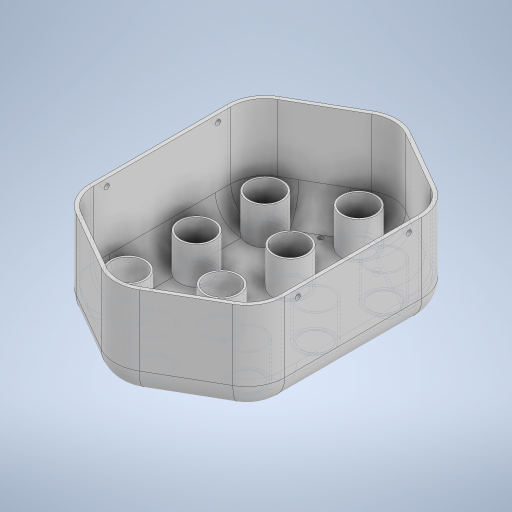
# Autodesk Inventor part: Caixa_10_amostras_v2
Saved by Autodesk Inventor 2024 (Build 280153000, 153)
## iProperties
Created: 2025-07-22
Part Number: Caixa_10_amostras_v2
Material: Generic
Document SubType Name: Modeling
Designer: Bruno
Density: 1 g/cm^3
Appearance: Default
Author: Bruno
Autodesk Inventor part; units mm, degrees
ref_plane "YZ Plane" through (0, 0, 0) normal (1, 0, 0) x (0, 1, 0)
ref_plane "XZ Plane" through (0, 0, 0) normal (0, 1, 0) x (-1, 0, 0)
ref_plane "XY Plane" through (0, 0, 0) normal (0, 0, 1) x (1, 0, 0)
sketch "Sketch1" plane through (0, 0, 0) normal (0, 1, 0) x (-1, 0, 0)
  line L0 (100, -100) -> (-100, -100)
  line L1 (-100, -100) -> (-100, 100)
  line L2 (-100, 100) -> (100, 100)
  line L3 (100, 100) -> (100, -100)
  line L4 (100, -100) -> (-100, 100)
  point P0 (0, 0)
  point P1 (0, 0)
  dimension "d0" = 200
  dimension "d1" = 200
  constraints: 10 end point, 2 parallel, 1 coincident, 1 horizontal, 1 midpoint, 1 perpendicular
  measures "d0" distance of L0.end L1.end
  measures "d1" distance of L0.start L0.end
extrude "Extrusion1" add sketch "Sketch1" along normal blind 2
sketch "Sketch2" plane through (0, 2, 0) normal (0, 1, 0) x (1, 0, 0)
  line L0 (100, 100) -> (-100, 100)
  line L1 (0, 100) -> (0, -100)
  line L2 (-100, -100) -> (100, -100)
  line L3 (100, -100) -> (100, 100)
  line L4 (100, 0) -> (-100, 0)
  line L5 (-100, 100) -> (-100, -100)
  circle A0 centre (0, -55.5) radius 18.5
  circle A1 centre (0, -55.5) radius 8.5
  circle A2 centre (0, -55.5) radius 17.5
  circle A3 centre (0, -55.5) radius 7.5
  circle A4 centre (0, -18.5) radius 7.5
  circle A5 centre (0, -18.5) radius 8.5
  circle A6 centre (0, -18.5) radius 17.5
  circle A7 centre (0, -18.5) radius 18.5
  circle A8 centre (0, 18.5) radius 7.5
  circle A9 centre (0, 18.5) radius 8.5
  circle A10 centre (0, 18.5) radius 17.5
  circle A11 centre (0, 18.5) radius 18.5
  circle A12 centre (0, 55.5) radius 7.5
  circle A13 centre (0, 55.5) radius 8.5
  circle A14 centre (0, 55.5) radius 17.5
  circle A15 centre (0, 55.5) radius 18.5
  circle A16 centre (-32.04294, -37) radius 7.5
  circle A17 centre (-32.04294, -37) radius 8.5
  circle A18 centre (-32.04294, -37) radius 17.5
  circle A19 centre (-32.04294, -37) radius 18.5
  circle A20 centre (-32.04294, 0) radius 7.5
  circle A21 centre (-32.04294, 0) radius 8.5
  circle A22 centre (-32.04294, 0) radius 17.5
  circle A23 centre (-32.04294, 0) radius 18.5
  circle A24 centre (-32.04294, 37) radius 7.5
  circle A25 centre (-32.04294, 37) radius 8.5
  circle A26 centre (-32.04294, 37) radius 17.5
  circle A27 centre (-32.04294, 37) radius 18.5
  circle A28 centre (32.05706, -37) radius 7.5
  circle A29 centre (32.05706, -37) radius 8.5
  circle A30 centre (32.05706, -37) radius 17.5
  circle A31 centre (32.05706, -37) radius 18.5
  circle A32 centre (32.05706, 0) radius 7.5
  circle A33 centre (32.05706, 0) radius 8.5
  circle A34 centre (32.05706, 0) radius 17.5
  circle A35 centre (32.05706, 0) radius 18.5
  circle A36 centre (32.05706, 37) radius 7.5
  circle A37 centre (32.05706, 37) radius 8.5
  circle A38 centre (32.05706, 37) radius 17.5
  circle A39 centre (32.05706, 37) radius 18.5
  point P0 (0, 0)
  point P1 (-32.04294, 18.5)
  point P2 (-16.02147, 27.75)
  point P3 (-16.02147, 46.25)
  point P4 (-16.02147, 9.25)
  point P5 (-32.04294, -18.5)
  point P6 (-16.02147, -9.25)
  point P7 (0, 37)
  point P8 (0, 0)
  point P9 (-16.02147, -27.75)
  point P10 (32.05706, 18.5)
  point P11 (32.05706, -18.5)
  dimension "d4" = 37
  dimension "d5" = 17
  dimension "d18" = 35
  dimension "d19" = 15
  dimension "d42" = 37
  dimension "d47" = 111
  dimension "d48" = 35
  dimension "d49" = 37
  dimension "d50" = 15
  dimension "d51" = 17
  dimension "d55" = 37
  dimension "d58" = 64.1
  constraints: 40 centre point, 30 coincident, 4 end point, 4 midpoint, 2 equal radius, 2 vertical, 1 horizontal, 1 point on line, 64 other
  measures "d4" diameter of A0
  measures "d5" diameter of A1
  measures "d18" diameter of A2
  measures "d19" diameter of A3
  measures "d42" distance of A3.centre A4.centre
  measures "d47" diameter of A0.centre L4
  measures "d48" diameter of A18
  measures "d49" diameter of A19
  measures "d50" diameter of A16
  measures "d51" diameter of A17
  measures "d55" distance of A16.centre A20.centre
  measures "d58" distance of A16.centre A28.centre
extrude "Extrusion2" cut sketch "Sketch2" against normal blind 0.1 contours A39 | A31 | A15 L1 A14 | L1 A14 A15 | A35 L4 A34 | L4 A34 A35 | A27 | A23 L4 A22 | L4 A22 A23 | A13 L1 A12 | L1 A12 A13 | A11 L1 A10 | L1 A10 A11 | A0 L1 A2 | L1 A2 A0 | A33 L4 A32 | L4 A32 A33 | A19 | A7 L1 A6 | L1 A6 A7 | A21 L4 A20 | L4 A20 A21 | A9 L1 A8 | L1 A8 A9 | A1 L1 A3 | L1 A3 A1 | A5 L1 A4 | L1 A4 A5 | A17 | A25 | A29 | A37
sketch "Sketch4" plane through (0, 2, 0) normal (0, 1, 0) x (1, 0, 0)
  arc A0 (-16.02147, 46.25) -> (-32.04294, 18.5) centre (-32.04294, 37) ccw
  line L0 (-41.29294, 53.02147) -> (-9.25, 71.52147)
  arc A1 (0, 37) -> (-16.02147, 46.25) centre (0, 55.5) ccw
  line L1 (9.246944, 71.523234) -> (41.304004, 53.023234)
  circle A2 centre (32.05706, 37) radius 18.5
  line L2 (50.55706, 37) -> (50.55706, -37)
  circle A3 centre (32.05706, -37) radius 18.5
  line L3 (41.304004, -53.023234) -> (9.246944, -71.523234)
  arc A4 (-16.02147, -46.25) -> (0, -37) centre (0, -55.5) ccw
  line L4 (-9.25, -71.52147) -> (-41.29294, -53.02147)
  line L5 (-50.54294, 37) -> (-50.54294, -37)
  arc A5 (-32.04294, -18.5) -> (-16.02147, -46.25) centre (-32.04294, -37) ccw
  line L6 (-100, 100) -> (-100, -100)
  line L7 (100, 100) -> (-100, 100)
  line L8 (100, -100) -> (100, 100)
  line L9 (-100, -100) -> (100, -100)
  point P0 (0, 0)
  point P1 (32.05706, 18.5)
  point P2 (32.05706, -18.5)
  constraints: 12 end point, 12 point on circle, 12 tangent
extrude "Extrusion4" cut sketch "Sketch4" against normal through all
sketch "Sketch6" plane through (0, 0, 0) normal (0, -1, 0) x (1, 0, 0)
  arc A0 (50.55706, 37) -> (41.304004, 53.023234) centre (32.05706, 37) ccw
  line L0 (41.304004, 53.023234) -> (9.246944, 71.523234)
  arc A1 (9.246944, 71.523234) -> (-9.25, 71.52147) centre (0, 55.5) ccw
  line L1 (-9.25, 71.52147) -> (-41.29294, 53.02147)
  arc A2 (-41.29294, 53.02147) -> (-50.54294, 37) centre (-32.04294, 37) ccw
  line L2 (-50.54294, 37) -> (-50.54294, -37)
  arc A3 (-50.54294, -37) -> (-41.29294, -53.02147) centre (-32.04294, -37) ccw
  line L3 (-41.29294, -53.02147) -> (-9.25, -71.52147)
  arc A4 (-9.25, -71.52147) -> (9.246944, -71.523234) centre (0, -55.5) ccw
  line L4 (9.246944, -71.523234) -> (41.304004, -53.023234)
  arc A5 (41.304004, -53.023234) -> (50.55706, -37) centre (32.05706, -37) ccw
  line L5 (50.55706, -37) -> (50.55706, 37)
  line L6 (10.246613, 73.255476) -> (42.303673, 54.755476)
  arc A6 (52.55706, 37) -> (42.303673, 54.755476) centre (32.05706, 37) ccw
  line L7 (52.55706, 37) -> (52.55706, -37)
  arc A7 (42.303673, -54.755476) -> (52.55706, -37) centre (32.05706, -37) ccw
  line L8 (42.303673, -54.755476) -> (10.246613, -73.255476)
  arc A8 (-10.25, -73.253521) -> (10.246613, -73.255476) centre (0, -55.5) ccw
  line L9 (-10.25, -73.253521) -> (-42.29294, -54.753521)
  arc A9 (-52.54294, -37) -> (-42.29294, -54.753521) centre (-32.04294, -37) ccw
  line L10 (-52.54294, -37) -> (-52.54294, 37)
  arc A10 (-42.29294, 54.753521) -> (-52.54294, 37) centre (-32.04294, 37) ccw
  line L11 (-42.29294, 54.753521) -> (-10.25, 73.253521)
  arc A11 (10.246613, 73.255476) -> (-10.25, 73.253521) centre (0, 55.5) ccw
  point P0 (0, 0)
  dimension "d65" = 2
  constraints: 12 end point, 12 point on circle, 6 centre point, 11 other
  measures "d65" distance between parallel lines of L6 L0
extrude "Extrusion6" add sketch "Sketch6" against normal blind 52
sketch "Sketch7" plane through (0, 1.9, 0) normal (0, 1, 0) x (1, 0, 0)
  arc A0 (-16.02147, -46.25) -> (-16.02147, -27.75) centre (-32.04294, -37) ccw
  arc A1 (-16.02147, -27.75) -> (-32.04294, -18.5) centre (-32.04294, -37) ccw
  arc A2 (-32.04294, -18.5) -> (-16.02147, -46.25) centre (-32.04294, -37) ccw
  circle A3 centre (-32.04294, -37) radius 17.5
  arc A4 (-16.02147, -9.25) -> (-16.02147, 9.25) centre (-32.04294, 0) ccw
  arc A5 (-16.02147, 9.25) -> (-32.04294, 18.5) centre (-32.04294, 0) ccw
  arc A6 (-32.04294, 18.5) -> (-32.04294, -18.5) centre (-32.04294, 0) ccw
  arc A7 (-32.04294, -18.5) -> (-16.02147, -9.25) centre (-32.04294, 0) ccw
  circle A8 centre (-32.04294, 0) radius 17.5
  arc A9 (-16.02147, 27.75) -> (-16.02147, 46.25) centre (-32.04294, 37) ccw
  arc A10 (-16.02147, 46.25) -> (-32.04294, 18.5) centre (-32.04294, 37) ccw
  arc A11 (-32.04294, 18.5) -> (-16.02147, 27.75) centre (-32.04294, 37) ccw
  circle A12 centre (-32.04294, 37) radius 17.5
  arc A13 (-16.02147, 46.25) -> (0, 37) centre (0, 55.5) ccw
  arc A14 (0, 37) -> (-16.02147, 46.25) centre (0, 55.5) ccw
  circle A15 centre (0, 55.5) radius 17.5
  arc A16 (-16.02147, 9.25) -> (0, 0) centre (0, 18.5) ccw
  arc A17 (0, 0) -> (0, 37) centre (0, 18.5) ccw
  arc A18 (0, 37) -> (-16.02147, 27.75) centre (0, 18.5) ccw
  arc A19 (-16.02147, 27.75) -> (-16.02147, 9.25) centre (0, 18.5) ccw
  circle A20 centre (0, 18.5) radius 17.5
  arc A21 (-16.02147, -9.25) -> (-16.02147, -27.75) centre (0, -18.5) ccw
  arc A22 (-16.02147, -27.75) -> (0, -37) centre (0, -18.5) ccw
  arc A23 (0, -37) -> (0, 0) centre (0, -18.5) ccw
  arc A24 (0, 0) -> (-16.02147, -9.25) centre (0, -18.5) ccw
  circle A25 centre (0, -18.5) radius 17.5
  arc A26 (-16.02147, -46.25) -> (0, -37) centre (0, -55.5) ccw
  arc A27 (0, -37) -> (-16.02147, -46.25) centre (0, -55.5) ccw
  circle A28 centre (0, -55.5) radius 17.5
  circle A29 centre (32.05706, -37) radius 18.5
  circle A30 centre (32.05706, -37) radius 17.5
  arc A31 (32.05706, -18.5) -> (32.05706, 18.5) centre (32.05706, 0) ccw
  arc A32 (32.05706, 18.5) -> (32.05706, -18.5) centre (32.05706, 0) ccw
  circle A33 centre (32.05706, 0) radius 17.5
  circle A34 centre (32.05706, 37) radius 18.5
  circle A35 centre (32.05706, 37) radius 17.5
  point P0 (0, 0)
  point P1 (32.05706, 18.5)
  point P2 (32.05706, 18.5)
  point P3 (32.05706, -18.5)
  point P4 (32.05706, -18.5)
  point P5 (0, 37)
  point P6 (0, 37)
  point P7 (0, 37)
  point P8 (0, 37)
  point P9 (-16.02147, 46.25)
  point P10 (-16.02147, 46.25)
  point P11 (-16.02147, 46.25)
  point P12 (-16.02147, 46.25)
  point P13 (-16.02147, 27.75)
  point P14 (-16.02147, 27.75)
  point P15 (-16.02147, 27.75)
  point P16 (-16.02147, 27.75)
  point P17 (0, -37)
  point P18 (0, -37)
  point P19 (0, -37)
  point P20 (0, -37)
  point P21 (-16.02147, -46.25)
  point P22 (-16.02147, -46.25)
  point P23 (-16.02147, -46.25)
  point P24 (-16.02147, -46.25)
  point P25 (-16.02147, -27.75)
  point P26 (-16.02147, -27.75)
  point P27 (-16.02147, -27.75)
  point P28 (-16.02147, -27.75)
  point P29 (-32.04294, -18.5)
  point P30 (-32.04294, -18.5)
  point P31 (-32.04294, -18.5)
  point P32 (-32.04294, -18.5)
  point P33 (0, 0)
  point P34 (0, 0)
  point P35 (0, 0)
  point P36 (0, 0)
  point P37 (-16.02147, -9.25)
  point P38 (-16.02147, -9.25)
  point P39 (-16.02147, -9.25)
  point P40 (-16.02147, -9.25)
  point P41 (-16.02147, 9.25)
  point P42 (-16.02147, 9.25)
  point P43 (-16.02147, 9.25)
  point P44 (-16.02147, 9.25)
  constraints: 2 other
extrude "Extrusion7" add sketch "Sketch7" along normal up to surface (0.1 mm away) contours A2 A1 A0 | A27 A26 | A21 A24 A23 A22 | A6 A5 A4 A7 | A10 A9 A11 | A16 A19 A18 A17 | A14 A13 | A29 | A34 | A32 A31
sketch "Sketch5" plane through (0, 2, -18.5) normal (0, 1, 0) x (1, 0, 0)
  circle A0 centre (-32.04294, 18.5) radius 8.5
  circle A1 centre (0, 37) radius 8.5
  circle A2 centre (32.05706, 18.5) radius 8.5
  circle A3 centre (0, 0) radius 8.5
  circle A4 centre (32.05706, -18.5) radius 8.5
  circle A5 centre (32.05706, -55.5) radius 8.5
  circle A6 centre (0, -37) radius 8.5
  circle A7 centre (0, -74) radius 8.5
  circle A8 centre (-32.04294, -55.5) radius 8.5
  circle A9 centre (-32.04294, -18.5) radius 8.5
  circle A10 centre (-32.04294, -55.5) radius 7.5
  circle A11 centre (-32.04294, -55.5) radius 9.5
  circle A12 centre (-32.04294, -18.5) radius 9.5
  circle A13 centre (-32.04294, 18.5) radius 9.5
  circle A14 centre (0, 0) radius 9.5
  circle A15 centre (0, 37) radius 9.5
  circle A16 centre (0, -37) radius 9.5
  circle A17 centre (0, -74) radius 9.5
  circle A18 centre (32.05706, -55.5) radius 9.5
  circle A19 centre (32.05706, -18.5) radius 9.5
  circle A20 centre (32.05706, 18.5) radius 7.5
  circle A21 centre (32.05706, 18.5) radius 9.5
  point P0 (0, -18.5)
  dimension "d68" = 1
  dimension "d69" = 1
  dimension "d70" = 1
  dimension "d71" = 1
  dimension "d72" = 1
  dimension "d73" = 1
  dimension "d74" = 1
  dimension "d75" = 1
  dimension "d76" = 1
  dimension "d77" = 1
  constraints: 10 centre point, 10 coincident
  measures "d68" radial gap between concentric circles of A11 A8
  measures "d69" radial gap between concentric circles of A12 A9
  measures "d70" radial gap between concentric circles of A13 A0
  measures "d71" radial gap between concentric circles of A16 A6
  measures "d72" radial gap between concentric circles of A14 A3
  measures "d73" radial gap between concentric circles of A15 A1
  measures "d74" radial gap between concentric circles of A17 A7
  measures "d75" radial gap between concentric circles of A18 A5
  measures "d76" radial gap between concentric circles of A19 A4
  measures "d77" radial gap between concentric circles of A21 A2
extrude "Extrusion5" add sketch "Sketch5" along normal blind 20 contours A11 | A12 | A13 | A14 | A15 | A16 | A17 | A18 | A19 | A21
fillet "Fillet2" radius 14 24 edges at (-48.0644, 2, 46.25) (-25.2715, 2, 62.2715) (-0.0018, 2, 74) (25.2755, 2, 62.2732) (48.0776, 2, 46.2515) (50.5571, 2, 0) (48.0776, 2, -46.2515) (25.2755, 2, -62.2732) (-0.0018, 2, -74) (-25.2715, 2, -62.2715) (-48.0644, 2, -46.25) (-50.5429, 2, 0) (49.8096, 0, 47.2517) (26.2751, 0, 64.0055) (-0.002, 0, 76) (-26.2715, 0, 64.0035) (-49.7965, 0, 47.25) (-52.5429, 0, 0) (-49.7965, 0, -47.25) (-26.2715, 0, -64.0035) (-0.002, 0, -76) (26.2751, 0, -64.0055) (49.8096, 0, -47.2517) (52.5571, 0, 0)
sketch "Sketch8" plane through (52.55706, 52, 37) normal (1, 0, 0) x (0, 0, -1)
  line L0 (37, 17.918603) -> (37, -112.555853)
  circle A0 centre (7, -3.9) radius 1.35
  line L1 (0, 0) -> (74, 0)
  circle A1 centre (67, -3.9) radius 1.35
  point P0 (37, -52)
  dimension "d81" = 2.7
  dimension "d82" = 60
  dimension "d83" = 3.9
  constraints: 2 centre point, 2 end point, 1 point on line, 1 symmetric about line, 1 vertical, 1 other
  measures "d81" diameter of A0
  measures "d82" diameter of A0.centre L0
  measures "d83" distance from line of L1 A0.centre
extrude "Extrusion8" cut sketch "Sketch8" against normal through all
sketch "Sketch9" plane through (0, 0, 0) normal (0, -1, 0) x (1, 0, 0)
  line L0 (-59.157848, 0) -> (59.157848, 0)
  line L1 (0, 117.504066) -> (0, -117.504066)
  circle A0 centre (-15, 50) radius 1.35
  circle A1 centre (15, 50) radius 1.35
  circle A2 centre (-15, -50) radius 1.35
  circle A3 centre (15, -50) radius 1.35
  point P0 (0, 0)
  point P1 (0, 0)
  dimension "d86" = 2.7
  dimension "d87" = 100
  dimension "d90" = 30
  constraints: 4 centre point, 4 end point, 3 symmetric about line, 2 midpoint, 1 coincident, 1 horizontal, 1 vertical, 3 other
  measures "d86" diameter of A0
  measures "d87" diameter of A0.centre L0
  measures "d90" diameter of A0.centre L1
extrude "Extrusion9" cut sketch "Sketch9" against normal through all
body "Solid1"
